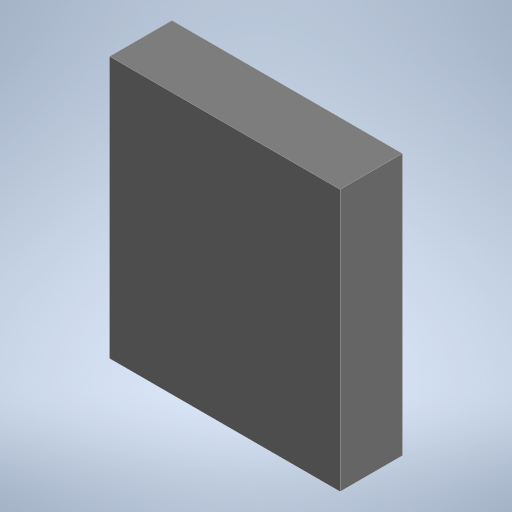
# Autodesk Inventor part: Spacer Bg
Saved by Autodesk Inventor 2024 (Build 280153000, 153)
## iProperties
Created: 2023-10-03
Part Number: Spacer Bg
Material: Generic
Document SubType Name: Modeling
Designer: flynf
Density: 1 g/cm^3
Appearance: Gray
Author: flynf
Autodesk Inventor part; units mm, degrees
ref_plane "YZ Plane" through (0, 0, 0) normal (1, 0, 0) x (0, 1, 0)
ref_plane "XZ Plane" through (0, 0, 0) normal (0, 1, 0) x (-1, 0, 0)
ref_plane "XY Plane" through (0, 0, 0) normal (0, 0, 1) x (1, 0, 0)
sketch "Sketch1" plane through (0, 0, 0) normal (0, 0, 1) x (1, 0, 0)
  line L0 (0, 0) -> (40.64, 0)
  line L1 (40.64, 0) -> (40.64, 53.34)
  line L2 (40.64, 53.34) -> (0, 53.34)
  line L3 (0, 53.34) -> (0, 0)
  dimension "d0" = 53.34
  dimension "d1" = 40.64
  constraints: 8 end point, 2 parallel, 1 horizontal, 1 perpendicular
  measures "d0" distance of L0.end L1.end
  measures "d1" distance of L1.end L2.end
extrude "Extrusion1" add sketch "Sketch1" along normal blind 12.7
sketch "Sketch2" plane through (40.64, 0, 0) normal (1, 0, 0) x (0, 0, -1)
  point P0 (0, 0)
sketch "Sketch3" plane through (40.64, 0, 0) normal (1, 0, 0) x (0, 0, -1)
  line L0 (0, 0) -> (-12.7, 0) projected
  line L1 (-12.7, 0) -> (-12.7, 53.34) projected
  line L2 (0, 0) -> (-12.7, 0)
  line L3 (-12.7, 0) -> (-12.7, 53.34)
  line L4 (-12.7, 53.34) -> (0, 53.34)
  line L5 (0, 53.34) -> (0, 0)
  constraints: 8 end point, 2 parallel, 1 horizontal, 1 perpendicular
extrude "Extrusion2" add sketch "Sketch3" along normal blind 6.35
body "Solid1"
